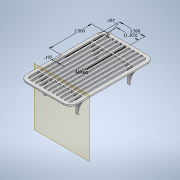
# Autodesk Inventor part: Part1
Saved by Autodesk Inventor 2021 (Build 250183000, 183)
## iProperties
Created: 2022-01-01
Part Number: Part1
Material: Generic
Document SubType Name: Modeling
Designer: Andrew
Density: 1 g/cm^3
Appearance: Default
Author: Andrew
Autodesk Inventor part; units mm, degrees
ref_plane "YZ Plane" through (0, 0, 0) normal (1, 0, 0) x (0, 1, 0)
ref_plane "XZ Plane" through (0, 0, 0) normal (0, 1, 0) x (-1, 0, 0)
sketch "Sketch2" plane through (0, 0, 0) normal (0, 1, 0) x (-1, 0, 0)
  line L0 (33.1, 0) -> (33.1, -53.5)
  line L1 (28.1, -58.5) -> (0, -58.5)
  line L2 (0, -58.5) -> (0, -63.5)
  line L3 (0, -63.5) -> (28.1, -63.5)
  line L4 (38.1, -53.5) -> (38.1, 0)
  arc A0 (28.1, -58.5) -> (33.1, -53.5) centre (28.1, -53.5) ccw
  arc A1 (28.1, -63.5) -> (38.1, -53.5) centre (28.1, -53.5) ccw
  line L5 (38.1, 0) -> (33.1, 0)
  line L6 (1.655, -58.5) -> (1.655, 0)
  line L7 (1.655, 0) -> (4.655, 0)
  line L8 (4.655, 0) -> (4.655, -58.5)
  line L9 (4.655, -58.5) -> (1.655, -58.5)
  point P0 (0, 0)
  dimension "d8" = 5
  dimension "d10" = 5
  dimension "d11" = 63.5
  dimension "d12" = 38.1
  dimension "d13" = 3
  dimension "d14" = 33.1
  dimension "d15" = 1.655
  constraints: 20 end point, 7 perpendicular, 4 point on circle, 4 point on line, 4 tangent, 2 centre point, 2 vertical, 1 collinear, 1 concentric, 1 horizontal
  measures "d8" radius of A0
  measures "d10" distance between parallel lines of L0 L4
  measures "d11" distance between parallel lines of L3 L5
  measures "d12" distance between parallel lines of L2 L4
  measures "d13" distance of L6.end L7.end
  measures "d14" distance between parallel lines of L2 L0
  measures "d15" distance between parallel lines of L2 L6
sketch "Sketch1" plane through (0, 0, 0) normal (0, 0, 1) x (1, 0, 0)
  arc A0 (11.43, -0.8621) -> (0, 0) centre (0, -76.2) ccw
  arc A1 (22.2231, -13.6401) -> (11.43, -0.8621) centre (9.525, -13.4184) ccw
  line L0 (22.2231, -13.6401) -> (22.0178, -25.4)
  line L1 (0, 17.64) -> (0, -91.84) construction
  line L2 (0, 0) -> (0, 2)
  line L3 (0, 2) -> (38.1, 2)
  line L4 (22.0178, -25.4) -> (27.0178, -25.4873)
  line L5 (38.1, 2) -> (38.1, 0)
  arc A2 (38.1, 0) -> (27.0178, -25.4873) centre (63.3247, -26.121) ccw
  dimension "d1" = 76.2
  dimension "d2" = 12.7
  dimension "d3" = 22.225
  dimension "d4" = 25.4
  dimension "d6" = 1
  dimension "d7" = 2
  dimension "d23" = 38.1
  dimension "d28" = 5
  constraints: 10 end point, 6 point on circle, 3 centre point, 2 perpendicular, 2 point on line, 2 tangent, 1 horizontal alignment, 1 vertical, 1 vertical alignment
  measures "d1" radius of A0
  measures "d2" radius of A1
  measures "d4" vertical distance of L0.end L2.start
  measures "d6" angle of L1 L0
  measures "d7" distance of L2.end L2.start
  measures "d23" distance of L2.end L3.end
  measures "d28" horizontal distance of L0.end L4.end
extrude "Extrusion1" add sketch "Sketch2" along normal blind 2 contours L5 L4 A1 L3 L2 L1 A0 L0
extrude "Extrusion2" add sketch "Sketch2" along normal blind 2 separate body contours L1 L6 L7 L8
pattern_linear "Rectangular Pattern1" count 5 spacing 6.31 along (-1, 0, 0) bodies 2
combine bodies "Combine1" operation type add bodies to combine 1 2
mirror "Mirror1" about plane through (0, 0, 0) normal (0, 0, 1) bodies 1
mirror "Mirror2" about plane through (0, 0, 0) normal (1, 0, 0) bodies 1
ref_plane "Work Plane1" through (0, 0, 38.1) normal (0, 0, 1) x (1, 0, 0)
extrude "Extrusion3" add sketch "Sketch1" along normal blind 2 from surface at 38.1 separate body
fillet "Fillet1" radius 1 8 edges at (5.7312, -0.2158, 40.1) (22.1204, -19.52, 40.1) (19.2271, -5.2234, 40.1) (30.024, -11.6414, 40.1) (19.2271, -5.2234, 38.1) (5.7312, -0.2158, 38.1) (22.1204, -19.52, 38.1) (30.024, -11.6414, 38.1)
mirror "Mirror3" about plane through (0, 0, 0) normal (1, 0, 0) bodies 3
mirror "Mirror4" about plane through (0, 0, 0) normal (0, 0, 1) bodies 3
combine bodies "Combine2" operation type add bodies to combine 1 3
equation "\"d23\" = d12"
equation "\"d22\" = 2 * d15 + d13"
body "Solid1"
